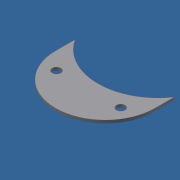
# Autodesk Inventor part: minimalEncoder
Saved by Autodesk Inventor 2014 SP2 (Build 180246200, 246)
## iProperties
Created: 2015-01-29
Part Number: minimalEncoder
Material: Generisch
Document SubType Name: Modeling
Designer: 4ndreas
Density: 1 g/cm^3
Appearance: Vorgabe
Author: 4ndreas
Autodesk Inventor part; units mm, degrees
ref_plane "YZ Plane" through (0, 0, 0) normal (1, 0, 0) x (0, 1, 0)
ref_plane "XZ Plane" through (0, 0, 0) normal (0, 1, 0) x (-1, 0, 0)
ref_plane "XY Plane" through (0, 0, 0) normal (0, 0, 1) x (1, 0, 0)
sketch "Skizze1" plane through (0, 0, 0) normal (0, 0, 1) x (1, 0, 0)
  circle A0 centre (0, 25) radius 18.5 construction
  circle A1 centre (11, 1.2967) radius 1.5 construction
  circle A2 centre (-11, 1.2967) radius 1.5 construction
  circle A3 centre (0, 0) radius 5.5 construction
  arc A4 (-13.7171, 6) -> (-17.4753, 0.6301) centre (-13.7171, 2) ccw construction
  arc A5 (-17.4753, 0.6301) -> (17.4753, 0.6301) centre (0, 7) ccw construction
  arc A6 (17.4753, 0.6301) -> (13.7171, 6) centre (13.7171, 2) ccw construction
  line L0 (-13.7171, 6) -> (13.7171, 6) construction
  arc A7 (-15.4919, -4) -> (15.4919, -4) centre (0, 7) ccw construction
  arc A8 (-13.2288, 2.1205) -> (13.2288, 2.1205) centre (0, 7) ccw construction
  line L1 (-13.2288, 2.1205) -> (-13.2288, 18) construction
  line L2 (13.2288, 18) -> (-13.2288, 18) construction
  arc A9 (-19, 7) -> (-9.4721, -9.4705) centre (0, 7) ccw construction
  line L3 (-9.4721, -9.4705) -> (-9.4721, -18.6052) construction
  spline S0 degree 3 poles (-9.4721, -18.6052) (-10.8029, -18.1851) (-12.1032, -17.6649) (-16.3725, -15.5421) (-18.9977, -13.5189) (-21.2475, -11.0387) knots -1.506344 -1.506344 -1.506344 -1.506344 -1.083379 -1.083379 -0.074726 -0.074726 -0.074726 -0.074726 construction
  spline S1 degree 3 poles (-21.2475, -11.0387) (-21.4119, -10.8574) (-21.5695, -10.6702) (-21.8699, -10.2854) (-22.0126, -10.0879) (-22.148, -9.8855) knots -0.146464 -0.146464 -0.146464 -0.146464 -0.073068 -0.073068 0 0 0 0 construction
  spline S2 degree 3 poles (-22.148, -9.8855) (-24.4473, -6.4457) (-26.1085, -2.5959) (-28.9023, 6.7167) (-29.697, 12.4269) (-30, 18) knots -2.91726 -2.91726 -2.91726 -2.91726 -1.674385 -1.674385 0 0 0 0 construction
  line L4 (-30, 18) -> (-19, 18) construction
  line L5 (-19, 18) -> (-19, 7) construction
  line L6 (19, 18) -> (30, 18) construction
  spline S3 degree 3 poles (30, 18) (29.697, 12.4269) (28.9023, 6.7167) (26.1085, -2.5959) (24.4473, -6.4457) (22.148, -9.8855) knots -2.986913 -2.986913 -2.986913 -2.986913 -1.313902 -1.313902 -0.072047 -0.072047 -0.072047 -0.072047 construction
  spline S4 degree 3 poles (22.148, -9.8855) (22.0126, -10.0879) (21.8699, -10.2854) (21.5695, -10.6702) (21.4119, -10.8574) (21.2475, -11.0387) knots -0.146464 -0.146464 -0.146464 -0.146464 -0.073396 -0.073396 0 0 0 0 construction
  spline S5 degree 3 poles (21.2475, -11.0387) (19.6253, -12.8271) (17.7977, -14.3889) (13.7909, -16.9377) (11.6878, -17.9058) (9.4721, -18.6052) knots -3.300626 -3.300626 -3.300626 -3.300626 -3.030289 -3.030289 -2.770214 -2.770214 -2.770214 -2.770214 construction
  line L7 (9.4721, -18.6052) -> (9.4721, -9.4705) construction
  arc A10 (9.4721, -9.4705) -> (19, 7) centre (0, 7) ccw construction
  line L8 (19, 7) -> (19, 18) construction
  spline S6 degree 3 poles (21.2475, 47.0387) (21.4119, 46.8574) (21.5695, 46.6702) (21.8699, 46.2854) (22.0126, 46.0879) (22.148, 45.8855) knots -0.146464 -0.146464 -0.146464 -0.146464 -0.073068 -0.073068 0 0 0 0 construction
  spline S7 degree 3 poles (22.148, 45.8855) (24.4473, 42.4457) (26.1085, 38.5959) (28.9023, 29.2833) (29.697, 23.5731) (30, 18) knots -2.91726 -2.91726 -2.91726 -2.91726 -1.674385 -1.674385 0 0 0 0 construction
  line L9 (30, 18) -> (19, 18) construction
  line L10 (19, 18) -> (19, 29) construction
  arc A11 (19, 29) -> (9.4721, 45.4705) centre (0, 29) ccw construction
  line L11 (9.4721, 45.4705) -> (9.4721, 54.6052) construction
  spline S8 degree 3 poles (9.4721, 54.6052) (10.8029, 54.1851) (12.1032, 53.6649) (16.3725, 51.5421) (18.9977, 49.5189) (21.2475, 47.0387) knots -1.506344 -1.506344 -1.506344 -1.506344 -1.083379 -1.083379 -0.074726 -0.074726 -0.074726 -0.074726 construction
  spline S9 degree 3 poles (-22.148, 45.8855) (-22.0126, 46.0879) (-21.8699, 46.2854) (-21.5695, 46.6702) (-21.4119, 46.8574) (-21.2475, 47.0387) knots -0.146464 -0.146464 -0.146464 -0.146464 -0.073396 -0.073396 0 0 0 0 construction
  spline S10 degree 3 poles (-21.2475, 47.0387) (-19.6253, 48.8271) (-17.7977, 50.3889) (-13.7909, 52.9377) (-11.6878, 53.9058) (-9.4721, 54.6052) knots -3.300626 -3.300626 -3.300626 -3.300626 -3.030289 -3.030289 -2.770214 -2.770214 -2.770214 -2.770214 construction
  line L12 (-9.4721, 54.6052) -> (-9.4721, 45.4705) construction
  arc A12 (-9.4721, 45.4705) -> (-19, 29) centre (0, 29) ccw construction
  line L13 (-19, 29) -> (-19, 18) construction
  line L14 (-19, 18) -> (-30, 18) construction
  spline S11 degree 3 poles (-30, 18) (-29.697, 23.5731) (-28.9023, 29.2833) (-26.1085, 38.5959) (-24.4473, 42.4457) (-22.148, 45.8855) knots -2.986913 -2.986913 -2.986913 -2.986913 -1.313902 -1.313902 -0.072047 -0.072047 -0.072047 -0.072047 construction
  arc A13 (-17, 7) -> (17, 7) centre (0, 7) ccw
  arc A14 (-17, 13.5436) -> (17, 13.5436) centre (0, 25) ccw
  line L15 (17, 7) -> (17, 13.5436)
  line L16 (-17, 7) -> (-17, 13.5436)
  line L17 (0, 29) -> (0, 0) construction
  arc A15 (-13.8612, -2.8421) -> (13.8612, -2.8421) centre (0, 7) ccw construction
  circle A16 centre (0, 25) radius 20.5 construction
  line L18 (13.2288, 2.1205) -> (13.2288, 18) projected
  point P0 (0, 0)
  dimension "d2" = 2
  dimension "d3" = 2
  constraints: 30 end point, 15 point on circle, 8 centre point, 8 vertical, 4 horizontal, 3 coincident, 3 tangent, 2 concentric, 2 parallel, 1 perpendicular, 1 point on line, 69 other
  measures "d2" radial gap between concentric circles of A0 A16
  measures "d3" radial gap between concentric circles of A15 A7
extrude "Extrusion1" add sketch "Skizze1" along normal blind 1
sketch "Skizze2" plane through (0, 0, 1) normal (0, 0, 1) x (1, 0, 0)
  arc A0 (-17, 7) -> (17, 7) centre (0, 7) ccw projected
  line L0 (17, 7) -> (17, 13.5436) projected
  arc A1 (-17, 13.5436) -> (17, 13.5436) centre (0, 25) ccw projected
  line L1 (-17, 13.5436) -> (-17, 7) projected
  line L2 (17, 13.5436) -> (-17, 13.5436) construction
  line L3 (-17, 13.5436) -> (-17, -10) construction
  line L4 (-17, -10) -> (17, -10) construction
  line L5 (17, -10) -> (17, 13.5436) construction
  circle A2 centre (0, 25) radius 20.5 construction
  line L6 (-17, 13.5436) -> (17, 36.4564) construction
  line L7 (17, 13.5436) -> (17, 36.4564) construction
  point P0 (0, 0)
  point P1 (11, 1.2967)
  point P2 (0, 0)
  point P3 (-11, 1.2967)
  dimension "d6" = 6
  dimension "d7" = 17
  dimension "d8" = 28
  dimension "d9" = 12.2469
  dimension "d10" = 13.5436
  dimension "d11" = 23.5436
  dimension "d12" = 34
  dimension "d13" = 9.0436
  dimension "d14" = 6.5436
  dimension "d15" = 11.4564
  dimension "d16" = 20.5
  dimension "d17" = 17
  dimension "d18" = 22.9129
  constraints: 12 end point, 2 parallel, 2 point on circle, 1 centre point, 1 coincident, 1 collinear, 1 concentric, 1 horizontal, 1 midpoint, 1 perpendicular, 1 point on line, 1 tangent
  measures "d6" distance from line of point (11, 1.297) L0
  measures "d7" distance from line of point (0, 0) L0
  measures "d8" distance from line of point (-11, 1.297) L0
  measures "d9" vertical distance of point (11, 1.297) L0.end
  measures "d10" vertical distance of point (0, 0) L0.end
  measures "d11" distance between parallel lines of L4 L2
  measures "d12" distance between parallel lines of L1 L0
  measures "d13" distance edge to line of A1 L2
  measures "d14" vertical distance of L0.end A0.centre
  measures "d15" vertical distance of L0.end A1.centre
  measures "d16" radius of A1
  measures "d17" radius of A0
  measures "d18" distance of L6.end L0.end
hole "Bohrung1" at (11, 1.2967, 1) at (-11, 1.2967, 1) direction (0, 0, -1) diameter 3 end through all
